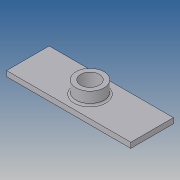
# Autodesk Inventor part: propstop
Saved by Autodesk Inventor 2019.4 (Build 234330000, 330)
## iProperties
Part Number: propstop
Material: GEDA Stahl
Document SubType Name: Modeling
Designer: Admin
Mass: 5.44398 g
Surface Area: 11.0178 cm^2
Volume: 0.692618 cm^3
Density: 7.86 g/cm^3
Appearance: GEDA Stahl A
Author: Admin
Gewicht: 0,005 kg
G_L: 0
G_H: 0
G_B: 0
InventorVersion: 2019.4
VAULT_Status: in Bearbeitung
Revision: -
Max. Breite: 0
Max. Höhe: 0
Max. Länge: 0
Max. Abmessungen: 0 x 0 x 0
Autodesk Inventor part; units mm, degrees
note: some values were not read from the file. Left out: dimensions or parameters whose unit could not be read.
ref_plane "YZ Plane" through (0, 0, 0) normal (1, 0, 0) x (0, 1, 0)
ref_plane "XZ Plane" through (0, 0, 0) normal (0, 1, 0) x (-1, 0, 0)
ref_plane "XY Plane" through (0, 0, 0) normal (0, 0, 1) x (1, 0, 0)
sketch "Skizze1" plane through (0, 0, 0) normal (0, 0, 1) x (1, 0, 0)
  line L0 (-17.5, -6) -> (17.5, -6)
  line L1 (17.5, -6) -> (17.5, 6)
  line L2 (17.5, 6) -> (-17.5, 6)
  line L3 (-17.5, 6) -> (-17.5, -6)
  line L4 (-17.5, -6) -> (17.5, 6) construction
  line L5 (17.5, -6) -> (-17.5, 6) construction
  point P0 (0, 0)
  dimension "d0" = 35
  dimension "d1" = 12
  constraints: 12 end point, 2 midpoint, 2 parallel, 1 horizontal, 1 perpendicular
  measures "d0" distance of L2.end L1.end
  measures "d1" distance of L1.end L0.end
extrude "Extrusion1" add sketch "Skizze1" along normal blind 1.5
sketch "Skizze2" plane through (0, 0, 1.5) normal (0, 0, 1) x (1, 0, 0)
  circle A0 centre (0, 0) radius 2.65
  dimension "d4" = 5.3
  constraints: 1 centre point, 1 coincident
  measures "d4" diameter of A0
extrude "Extrusion2" cut sketch "Skizze2" against normal blind 1.5
sketch "Skizze3" plane through (0, 0, 1.5) normal (0, 0, 1) x (1, 0, 0)
  circle A0 centre (0, 0) radius 3.95
  circle A1 centre (0, 0) radius 2.65 projected
  dimension "d7" = 7.9
  constraints: 1 centre point, 1 coincident
  measures "d7" diameter of A0
extrude "Extrusion3" add sketch "Skizze3" along normal blind 3.5
fillet "Rundung1" radius 0.5 1 edges at (-3.95, 0, 1.5)
equation "\"G_L\" = 0"
equation "\"G_H\" = 0"
equation "\"G_B\" = 0"
